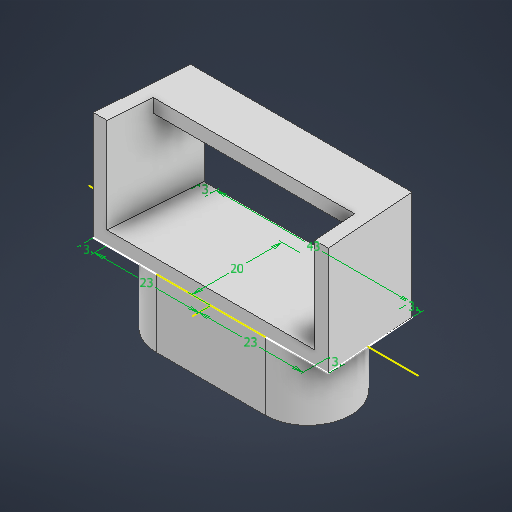
# Autodesk Inventor part: 카메라 상단
Saved by Autodesk Inventor 2026.2 (Build 302298000, 298)
## iProperties
Created: 2026-01-04
Part Number: 카메라 상단
Material: 일반
Document SubType Name: Modeling
Designer: PC
Density: 1 g/cm^3
Appearance: 기본값
Author: PC
Autodesk Inventor part; units mm, degrees
ref_plane "YZ Plane" through (0, 0, 0) normal (1, 0, 0) x (0, 1, 0)
ref_plane "XZ Plane" through (0, 0, 0) normal (0, 1, 0) x (-1, 0, 0)
ref_plane "XY Plane" through (0, 0, 0) normal (0, 0, 1) x (1, 0, 0)
sketch "스케치1" plane through (0, 0, 0) normal (0, 1, 0) x (-1, 0, 0)
  circle A0 centre (12, 0) radius 5.5
  circle A1 centre (-12, 0) radius 5.5
  line L0 (30.1, 0) -> (-30.1, 0) projected
  line L1 (12, 0) -> (-12, 0) construction
  line L2 (12, 9.5) -> (-12, 9.5)
  line L3 (-12, -9.5) -> (12, -9.5)
  arc A2 (12, -9.5) -> (12, 9.5) centre (12, 0) ccw
  arc A3 (-12, 9.5) -> (-12, -9.5) centre (-12, 0) ccw
  point P0 (0, 0)
  point P1 (0, 0)
  dimension "d0" = 11
  dimension "d1" = 11
  dimension "d2" = 12
  dimension "d3" = 12
  dimension "d4" = 4
  constraints: 8 end point, 4 centre point, 4 point on circle, 4 tangent, 2 point on line, 1 collinear, 1 midpoint, 1 parallel
  measures "d0" diameter of A0
  measures "d1" diameter of A1
  measures "d2" distance of L1.start point (0, 0)
  measures "d3" distance of point (0, 0) L1.end
  measures "d4" radial gap between concentric circles of A3 A1
extrude "돌출1" add sketch "스케치1" along normal blind 15 contours L0 A2 L3 A3 A1 A0 | A0 L0 A1 A3 L2 A2
sketch "스케치2" plane through (0, 15, 0) normal (0, 1, 0) x (1, 0, 0)
  line L0 (-12, -9.5) -> (12, -9.5) projected
  line L1 (0, -9.5) -> (-23, -9.5)
  line L2 (0, -9.5) -> (23, -9.5)
  line L3 (-21.5, 10.5) -> (21.5, 10.5)
  line L4 (-36.4, 0) -> (36.4, 0) projected
  line L5 (0, 14.5) -> (0, -13.5) projected
  line L6 (0, -9.5) -> (0, 10.5)
  line L7 (-21.5, 10.5) -> (-23, -9.5)
  line L8 (21.5, 10.5) -> (23, -9.5)
  line L9 (-23, -9.5) -> (-26, -9.5)
  line L10 (23, -9.5) -> (26, -9.5)
  line L11 (-21.5, 10.5) -> (-24.5, 10.5)
  line L12 (-24.5, 10.5) -> (-26, -9.5)
  line L13 (21.5, 10.5) -> (24.5, 10.5)
  line L14 (24.5, 10.5) -> (26, -9.5)
  point P0 (0, 0)
  dimension "d7" = 23
  dimension "d8" = 23
  dimension "d9" = 43
  dimension "d10" = 20
  dimension "d11" = 3
  dimension "d12" = 3
  dimension "d13" = 3
  dimension "d14" = 3
  constraints: 24 end point, 4 horizontal, 2 collinear, 2 midpoint, 2 point on line
  measures "d7" distance of L1.start L1.end
  measures "d8" distance of L1.start L2.end
  measures "d9" distance of L3.start L3.end
  measures "d10" distance of L6.end L1.start
  measures "d11" distance of L1.end L9.end
  measures "d12" distance of L2.end L10.end
  measures "d13" distance of L3.start L11.end
  measures "d14" distance of L3.end L13.end
extrude "돌출2" add sketch "스케치2" along normal blind 3
sketch "스케치3" plane through (0, 18, 0) normal (0, 1, 0) x (1, 0, 0)
  line L0 (-21.5, 10.5) -> (-23, -9.5) projected
  line L1 (21.5, 10.5) -> (23, -9.5) projected
  line L2 (-26, -9.5) -> (26, -9.5) projected
  line L3 (26, -9.5) -> (24.5, 10.5) projected
  line L4 (24.5, 10.5) -> (-24.5, 10.5) projected
  line L5 (-24.5, 10.5) -> (-26, -9.5) projected
  point P0 (0, 0)
  point P1 (23, -9.5)
  point P2 (-23, -9.5)
extrude "돌출3" add sketch "스케치3" along normal blind 18 contours L0 L2 L5 L4 | L4 L3 L2 L1
sketch "스케치4" plane through (0, 36, 0) normal (0, 1, 0) x (1, 0, 0)
  line L0 (23, -9.5) -> (21.5, 10.5) projected
  line L1 (21.5, 10.5) -> (-21.5, 10.5) projected
  line L2 (-21.5, 10.5) -> (-23, -9.5) projected
  line L3 (-23, -9.5) -> (23, -9.5) projected
  line L4 (-22.2875, 0) -> (22.2875, 0)
  line L5 (-26, -9.5) -> (-23, -9.5) projected
  line L6 (-23, -9.5) -> (-21.5, 10.5) projected
  line L7 (-21.5, 10.5) -> (-24.5, 10.5) projected
  line L8 (-24.5, 10.5) -> (-26, -9.5) projected
  line L9 (24.5, 10.5) -> (21.5, 10.5) projected
  line L10 (21.5, 10.5) -> (23, -9.5) projected
  line L11 (23, -9.5) -> (26, -9.5) projected
  line L12 (26, -9.5) -> (24.5, 10.5) projected
  point P0 (0, 0)
  point P1 (0, 0)
  constraints: 2 end point, 2 point on line, 1 coincident, 1 horizontal, 1 midpoint
extrude "돌출4" add sketch "스케치4" along normal blind 3 contours L0 L9 L12 L11 | L4 L2 L1 L0 | L5 L8 L7 L2
